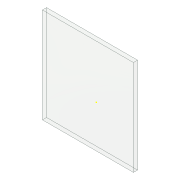
# Autodesk Inventor part: Plexiglass
Saved by Autodesk Inventor 2017 (Build 210142000, 142)
## iProperties
Created: 2018-11-30
Part Number: Plexiglass
Material: Glass
Document SubType Name: Modeling
Designer: jpb34
Mass: 282.441 g
Surface Area: 444.354 cm^2
Volume: 129.56 cm^3
Density: 2.18 g/cm^3
Appearance: Clear
Author: jpb34
Autodesk Inventor part; units mm, degrees
ref_plane "YZ Plane" through (0, 0, 0) normal (1, 0, 0) x (0, 1, 0)
ref_plane "XZ Plane" through (0, 0, 0) normal (0, 1, 0) x (-1, 0, 0)
ref_plane "XY Plane" through (0, 0, 0) normal (0, 0, 1) x (1, 0, 0)
sketch "Sketch1" plane through (0, 0, 0) normal (0, 0, 1) x (1, 0, 0)
  point P0 (0, 0)
sketch "Sketch2" plane through (0, 0, 0) normal (0, 0, 1) x (1, 0, 0)
  line L0 (-76.5648, 87.4558) -> (63.1352, 87.4558)
  line L1 (63.1352, 87.4558) -> (63.1352, -58.5942)
  line L2 (63.1352, -58.5942) -> (-76.5648, -58.5942)
  line L3 (-76.5648, -58.5942) -> (-76.5648, 87.4558)
  point P0 (0, 0)
  dimension "d0" = 139.7
  dimension "d1" = 146.05
  dimension "d2" = 63.1352
  dimension "d3" = 87.4558
  constraints: 8 end point, 2 parallel, 1 horizontal, 1 perpendicular
  measures "d0" distance of L0.start L0.end
  measures "d1" distance of L0.end L1.end
  measures "d2" distance from line of point (0, 0) L1
  measures "d3" distance from line of point (0, 0) L0
extrude "Extrusion1" add sketch "Sketch2" along normal blind 6.35
body "Solid1"
